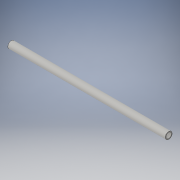
# Autodesk Inventor part: cAxelPVC3_4inchSchedule40
Saved by Autodesk Inventor 2016 SP1 (Build 200210100, 210)
## iProperties
Created: 2016-01-12
Part Number: cAxelPVC3_4inchSchedule40
Material: Generic
Document SubType Name: Modeling
Designer: steele
Density: 1 g/cm^3
Appearance: Default
Author: steele
Autodesk Inventor part; units mm, degrees
ref_plane "YZ Plane" through (0, 0, 0) normal (1, 0, 0) x (0, 1, 0)
ref_plane "XZ Plane" through (0, 0, 0) normal (0, 1, 0) x (-1, 0, 0)
ref_plane "XY Plane" through (0, 0, 0) normal (0, 0, 1) x (1, 0, 0)
sketch "Sketch3" plane through (0, 0, 0) normal (1, 0, 0) x (0, 1, 0)
  circle A0 centre (0, 0) radius 10.4648
  circle A1 centre (0, 0) radius 13.335
  dimension "d10" = 26.67
  dimension "d11" = 20.9296
  constraints: 2 centre point, 2 coincident
  measures "d10" diameter of A1
  measures "d11" diameter of A0
extrude "Extrusion3" add sketch "Sketch3" along normal blind 609.6
equation "\"d10\" = cArmOutsideDiam"
equation "\"d11\" = cArmInsideDiam"
equation "\"d12\" = cArmLength"
equation "\"catapultArmWallThickness\" = 1.5875"
equation "\"catapultArmWidth\" = 50.8"
equation "\"catapultArmLength\" = 1219.2"
equation "\"catapultArmAxelHoleDaim\" = 12.7"
equation "\"catapultArmHoleDistanceFromEnd\" = 381"
equation "\"cArmInsideDiam\" = 20.9296"
equation "\"cArmOutsideDiam\" = 26.67"
equation "\"cArmLength\" = 609.6"
body "Solid2"
